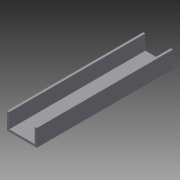
# Autodesk Inventor part: angle channel
Saved by Autodesk Inventor 2014 SP1 (Build 180222100, 222)
## iProperties
Created: 2015-02-04
Part Number: angle channel
Material: Generic
Document SubType Name: Modeling
Designer: degan
Density: 1 g/cm^3
Appearance: Default
Author: degan
Autodesk Inventor part; units mm, degrees
ref_plane "YZ Plane" through (0, 0, 0) normal (1, 0, 0) x (0, 1, 0)
ref_plane "XZ Plane" through (0, 0, 0) normal (0, 1, 0) x (-1, 0, 0)
ref_plane "XY Plane" through (0, 0, 0) normal (0, 0, 1) x (1, 0, 0)
sketch "Sketch1" plane through (0, 0, 0) normal (0, 0, 1) x (1, 0, 0)
  line L0 (24.1101, 25.4) -> (24.1101, 0)
  line L1 (24.1101, 0) -> (-20.3399, 0)
  line L2 (-20.3399, 0) -> (-20.3399, 25.4)
  line L3 (-17.1649, 25.4) -> (-17.1649, 3.175)
  line L4 (-17.1649, 3.175) -> (20.9351, 3.175)
  line L5 (20.9351, 3.175) -> (20.9351, 25.4)
  line L6 (-20.3399, 25.4) -> (-17.1649, 25.4)
  line L7 (24.1101, 25.4) -> (20.9351, 25.4)
  point P0 (0, 0)
  dimension "d0" = 44.45
  dimension "d1" = 25.4
  dimension "d2" = 3.175
  constraints: 16 end point, 3 equal length, 1 perpendicular, 2 other
  measures "d0" distance of L0.end L1.end
  measures "d1" distance of L1.end L2.end
  measures "d2" distance between parallel lines of L0 L5
extrude "Extrusion1" add sketch "Sketch1" against normal blind 203.2
body "Solid1"
